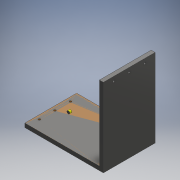
# Autodesk Inventor part: ConcreteFormwork
Saved by Autodesk Inventor 2016 (Build 200138000, 138)
## iProperties
Created: 2015-06-04
Part Number: ConcreteFormwork
Material: Wood (Birch)
Document SubType Name: Modeling
Designer: krosie
Density: 0.55 g/cm^3
Appearance: Birch - Natural Polished
Author: krosie
Autodesk Inventor part; units mm, degrees
ref_plane "YZ Plane" through (0, 0, 0) normal (1, 0, 0) x (0, 1, 0)
ref_plane "XZ Plane" through (0, 0, 0) normal (0, 1, 0) x (-1, 0, 0)
ref_plane "XY Plane" through (0, 0, 0) normal (0, 0, 1) x (1, 0, 0)
sketch "Sketch1" plane through (0, 0, 0) normal (0, 1, 0) x (-1, 0, 0)
  line L0 (-156.7682, 187.5) -> (-156.7682, -172.5)
  line L1 (-156.7682, 187.5) -> (203.2318, 187.5) construction
  line L2 (-156.7682, -172.5) -> (203.2318, -172.5)
  line L3 (-149.2682, 187.5) -> (-119.2682, 187.5) construction
  point P0 (0, 0)
  dimension "d0" = 360
  dimension "d1" = 90
  dimension "d2" = 360
  constraints: 8 end point, 2 horizontal, 2 perpendicular, 1 point on line, 1 vertical
  measures "d0" distance of L0.start L0.end
  measures "d1" angle of L0 L1
  measures "d2" distance of L0.end L2.end
surface extrude "ExtrusionSrf1" sketch "Sketch1" along normal blind 250 shown yes curves L0 L2
thicken "Thicken1" operation new thickness 19 both sides no extend neighbours no toward (1, 0, 0) faces at (156.7682, 83.3333, 67.5) (36.7682, 83.3333, -172.5)
hole "Hole1" at (-183.2318, 200, -172.5) direction (0, 0, -1) diameter 10 end through all
hole "Hole2" at (-183.2318, 125, -172.5) direction (0, 0, -1) diameter 10 end through all
hole "Hole3" at (-183.2318, 50, -172.5) direction (0, 0, -1) diameter 10 end through all
hole "Hole4" at (156.7682, 200, 167.5) direction (1, 0, 0) diameter 10 end through all
hole "Hole5" at (156.7682, 125, 167.5) direction (1, 0, 0) diameter 10 end through all
hole "Hole6" at (156.7682, 50, 167.5) direction (1, 0, 0) diameter 10 end through all
sketch "Sketch3" plane through (-203.2318, 0, -191.5) normal (0, -1, 0) x (1, 0, 0)
  line L0 (360, 379) -> (360, 19) projected
  line L1 (360, 19) -> (0, 19) projected
  circle A0 centre (210, 169) radius 6.9816
  point P0 (203.2318, 191.5)
  dimension "d75" = 150
  dimension "d76" = 150
  constraints: 1 centre point
  measures "d75" distance from line of L0 A0.centre
  measures "d76" distance from line of L1 A0.centre
extrude "Extrusion1" add sketch "Sketch3" against normal blind 10 separate body
body "Solid1"
body "Srf1"
body "Solid2"
